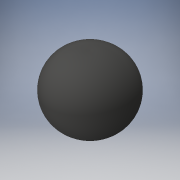
# Autodesk Inventor part: balle
Saved by Autodesk Inventor 2016 (Build 200138000, 138)
## iProperties
Created: 2016-01-25
Part Number: balle
Material: Generic
Document SubType Name: Modeling
Designer: ares-b02
Density: 1 g/cm^3
Appearance: Rubber - Black
Author: ares-b02
Autodesk Inventor part; units mm, degrees
ref_plane "YZ Plane" through (0, 0, 0) normal (1, 0, 0) x (0, 1, 0)
ref_plane "XZ Plane" through (0, 0, 0) normal (0, 1, 0) x (-1, 0, 0)
ref_plane "XY Plane" through (0, 0, 0) normal (0, 0, 1) x (1, 0, 0)
sketch "Sketch1" plane through (0, 0, 0) normal (0, 0, 1) x (1, 0, 0)
  arc A0 (-9.7944, 261.887) -> (-9.7944, -244.1058) centre (-32.3513, 8.8906) ccw
  line L0 (-9.7944, 261.887) -> (-9.7944, -244.1058)
  dimension "d1" = 254
  dimension "d1" = 254
  constraints: 2 end point, 2 point on circle, 1 centre point, 1 vertical
  measures "d1" radius of A0
revolve "Revolution1" add sketch "Sketch1" angle 360 about axis through (-9.7944, 261.887, 0) along (0, -1, 0)
body "Solid1"
